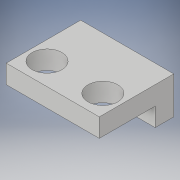
# Autodesk Inventor part: TensionerPlate4
Saved by Autodesk Inventor 2017 (Build 210142000, 142)
## iProperties
Created: 2018-05-12
Part Number: TensionerPlate4
Material: Generic
Document SubType Name: Modeling
Designer: User
Density: 1 g/cm^3
Appearance: Default
Author: User
Autodesk Inventor part; units mm, degrees
ref_plane "YZ Plane" through (0, 0, 0) normal (1, 0, 0) x (0, 1, 0)
ref_plane "XZ Plane" through (0, 0, 0) normal (0, 1, 0) x (-1, 0, 0)
ref_plane "XY Plane" through (0, 0, 0) normal (0, 0, 1) x (1, 0, 0)
sketch "Sketch1" plane through (0, 0, 0) normal (1, 0, 0) x (0, 1, 0)
  line L0 (0, 0) -> (12.7, 0)
  line L1 (12.7, 0) -> (12.7, -25.4)
  line L2 (12.7, -25.4) -> (0, -25.4)
  line L3 (0, -25.4) -> (0, 0)
  line L4 (0, 0) -> (6.35, 0)
  line L5 (6.35, 0) -> (6.35, -19.05)
  line L6 (6.35, -19.05) -> (0, -19.05)
  line L7 (0, -19.05) -> (0, 0)
  dimension "d0" = 12.7
  dimension "d1" = 25.4
  dimension "d2" = 6.35
  dimension "d3" = 6.35
  constraints: 16 end point, 4 parallel, 2 horizontal, 2 perpendicular
  measures "d0" distance of L1.end L2.end
  measures "d1" distance of L0.end L1.end
  measures "d2" distance between parallel lines of L5 L1
  measures "d3" distance between parallel lines of L2 L6
extrude "Extrusion1" add sketch "Sketch1" along normal blind 31.75 contours L0 L1 L2 L3 L6 L5
sketch "Sketch2" plane through (0, 12.7, 0) normal (0, 1, 0) x (1, 0, 0)
  line L0 (0, 25.4) -> (0, 0) projected
  line L1 (0, 0) -> (31.75, 0) projected
  line L2 (31.75, 25.4) -> (31.75, 0) projected
  line L3 (0, 25.4) -> (31.75, 25.4) projected
  point P0 (6.35, 7.562)
  point P1 (25.4, 7.562)
  dimension "d6" = 31.75
  dimension "d7" = 6.35
  dimension "d8" = 6.35
  measures "d6" distance of L0.end L1.end
  measures "d7" distance from line of L0 point (6.35, 7.562)
  measures "d8" distance from line of L2 point (25.4, 7.562)
hole "Hole1" at (6.35, 12.7, -7.562) at (25.4, 12.7, -7.562) direction (0, -1, 0) diameter 10.16 depth 22.9362 tip angle 118
equation "\"d8\" = d7"
body "Solid1"
